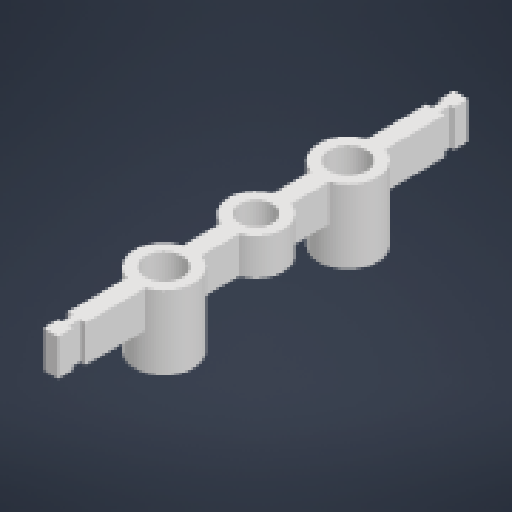
# Autodesk Inventor part: Leg_rod
Saved by Autodesk Inventor 2026 (Build 300175050, 175E)
## iProperties
Created: 2026-05-02
Part Number: Leg_rod
Material: Generic
Document SubType Name: Modeling
Designer: sniel
Density: 1 g/cm^3
Appearance: Default
Author: sniel
Autodesk Inventor part; units mm, degrees
ref_plane "YZ Plane" through (0, 0, 0) normal (1, 0, 0) x (0, 1, 0)
ref_plane "XZ Plane" through (0, 0, 0) normal (0, 1, 0) x (-1, 0, 0)
ref_plane "XY Plane" through (0, 0, 0) normal (0, 0, 1) x (1, 0, 0)
sketch "Sketch1" plane through (0, 0, 0) normal (0, 1, 0) x (-1, 0, 0)
  line L0 (16.7626, -83.8715) -> (19.7626, -83.8715) projected
  line L1 (19.7626, -83.8715) -> (19.7626, -85.3715) projected
  line L2 (19.7626, -85.3715) -> (10.7873, -88.3968) projected
  line L3 (10.7873, -88.3968) -> (7.7622, -97.3718) projected
  line L4 (7.7622, -97.3718) -> (6.2622, -97.3718) projected
  line L5 (6.2622, -97.3718) -> (6.2622, -94.3718) projected
  line L6 (6.2622, -94.3718) -> (7.2622, -94.3718) projected
  line L7 (7.2622, -94.3718) -> (7.2622, -90.3718) projected
  line L8 (7.2622, -90.3718) -> (3.2622, -90.3718) projected
  line L9 (3.2622, -90.3718) -> (3.2622, -94.3718) projected
  line L10 (3.2622, -94.3718) -> (4.2622, -94.3718) projected
  line L11 (4.2622, -94.3718) -> (4.2622, -97.3718) projected
  line L12 (4.2622, -97.3718) -> (2.7622, -97.3718) projected
  line L13 (2.7622, -97.3718) -> (-1.3715, -85.1077) projected
  arc A0 (7.4979, -76.2381) -> (-1.3715, -85.1077) centre (5.2622, -82.8718) ccw projected
  line L14 (7.4979, -76.2381) -> (19.7626, -80.3715) projected
  line L15 (19.7626, -80.3715) -> (19.7626, -81.8715) projected
  line L16 (19.7626, -81.8715) -> (16.7626, -81.8715) projected
  line L17 (16.7626, -81.8715) -> (16.7626, -80.8715) projected
  line L18 (16.7626, -80.8715) -> (12.7626, -80.8715) projected
  line L19 (12.7626, -80.8715) -> (12.7626, -84.8715) projected
  line L20 (12.7626, -84.8715) -> (16.7626, -84.8715) projected
  line L21 (16.7626, -84.8715) -> (16.7626, -83.8715) projected
  line L22 (6.3619, -198.0335) -> (6.3619, -195.0335) projected
  line L23 (6.3619, -195.0335) -> (7.8619, -195.0335) projected
  line L24 (7.8619, -195.0335) -> (10.8872, -204.0087) projected
  line L25 (10.8872, -204.0087) -> (19.8622, -207.0338) projected
  line L26 (19.8622, -207.0338) -> (19.8622, -208.5338) projected
  line L27 (19.8622, -208.5338) -> (16.8622, -208.5338) projected
  line L28 (16.8622, -208.5338) -> (16.8622, -207.5338) projected
  line L29 (16.8622, -207.5338) -> (12.8622, -207.5338) projected
  line L30 (12.8622, -207.5338) -> (12.8622, -211.5338) projected
  line L31 (12.8622, -211.5338) -> (16.8622, -211.5338) projected
  line L32 (16.8622, -211.5338) -> (16.8622, -210.5338) projected
  line L33 (16.8622, -210.5338) -> (19.8622, -210.5338) projected
  line L34 (19.8622, -210.5338) -> (19.8622, -212.0338) projected
  line L35 (19.8622, -212.0338) -> (7.5981, -216.1675) projected
  arc A1 (-1.2715, -207.2981) -> (7.5981, -216.1675) centre (5.3622, -209.5338) ccw projected
  line L36 (-1.2715, -207.2981) -> (2.8619, -195.0335) projected
  line L37 (2.8619, -195.0335) -> (4.3619, -195.0335) projected
  line L38 (4.3619, -195.0335) -> (4.3619, -198.0335) projected
  line L39 (4.3619, -198.0335) -> (3.3619, -198.0335) projected
  line L40 (3.3619, -198.0335) -> (3.3619, -202.0335) projected
  line L41 (3.3619, -202.0335) -> (7.3619, -202.0335) projected
  line L42 (7.3619, -202.0335) -> (7.3619, -198.0335) projected
  line L43 (7.3619, -198.0335) -> (6.3619, -198.0335) projected
  line L44 (2.7622, -97.3718) -> (2.8619, -195.0335)
  line L45 (7.8619, -195.0335) -> (7.7622, -97.3718)
  line L46 (2.812, -146.2026) -> (7.812, -146.2026)
  circle A2 centre (5.312, -146.2026) radius 4.5
  circle A3 centre (5.312, -146.2026) radius 7.5
  point P0 (0, 0)
  point P1 (7.8048, -139.129)
  point P2 (2.8048, -139.1341)
  point P3 (2.8193, -153.2762)
  point P4 (7.8193, -153.2711)
  dimension "d8" = 9
  dimension "d9" = 15
  constraints: 6 end point, 3 midpoint, 2 centre point, 1 coincident, 1 parallel
  measures "d8" diameter of A2
  measures "d9" diameter of A3
extrude "Extrusion1" add sketch "Sketch1" along normal blind 10 contours L45 A3 L44 L12 L11 L10 L9 L8 L7 L6 L5 L4 | A3 L45 A2 | L45 A2 L44 A3 | L44 A2 A3 | A3 L44 A2 L45 | L45 L23 L22 L43 L42 L41 L40 L39 L38 L37 L44 A3
sketch "Sketch2" plane through (0, 0, 0) normal (0, -1, 0) x (1, 0, 0)
  line L0 (-4.3619, -198.0335) -> (-3.3619, -198.0335)
  line L1 (-4.3619, -195.0335) -> (-4.3619, -198.0335)
  line L2 (-2.8619, -195.0335) -> (-4.3619, -195.0335)
  line L3 (-2.7622, -97.3718) -> (-2.8619, -195.0335)
  line L4 (-4.2622, -97.3718) -> (-2.7622, -97.3718)
  line L5 (-4.2622, -94.3718) -> (-4.2622, -97.3718)
  line L6 (-3.2622, -94.3718) -> (-4.2622, -94.3718)
  line L7 (-3.2622, -90.3718) -> (-3.2622, -94.3718)
  line L8 (-7.2622, -90.3718) -> (-3.2622, -90.3718)
  line L9 (-7.2622, -94.3718) -> (-7.2622, -90.3718)
  line L10 (-6.2622, -94.3718) -> (-7.2622, -94.3718)
  line L11 (-6.2622, -97.3718) -> (-6.2622, -94.3718)
  line L12 (-7.7622, -97.3718) -> (-6.2622, -97.3718)
  line L13 (-7.8619, -195.0335) -> (-7.7622, -97.3718)
  line L14 (-6.3619, -195.0335) -> (-7.8619, -195.0335)
  line L15 (-6.3619, -198.0335) -> (-6.3619, -195.0335)
  line L16 (-7.3619, -198.0335) -> (-6.3619, -198.0335)
  line L17 (-7.3619, -202.0335) -> (-7.3619, -198.0335)
  line L18 (-3.3619, -202.0335) -> (-7.3619, -202.0335)
  line L19 (-3.3619, -198.0335) -> (-3.3619, -202.0335)
  line L20 (-7.812, -146.2026) -> (-2.812, -146.2026)
  line L21 (-6.2622, -97.3718) -> (-4.2622, -97.3718)
  line L22 (-5.312, -146.2026) -> (-5.312, -121.2026)
  line L23 (-5.312, -146.2026) -> (-5.312, -171.2026)
  circle A0 centre (-5.312, -171.2026) radius 8
  circle A1 centre (-5.312, -121.2026) radius 8
  point P0 (0, 0)
  dimension "d2" = 25
  dimension "d3" = 25
  dimension "d4" = 16
  dimension "d5" = 16
  constraints: 48 end point, 3 midpoint, 2 centre point, 2 coincident, 2 vertical, 1 horizontal
  measures "d2" distance of L22.start L22.end
  measures "d3" distance of L22.start L23.end
  measures "d4" diameter of A0
  measures "d5" diameter of A1
extrude "Extrusion2" add sketch "Sketch2" along normal mid plane 20 contours A0 L13 L3 | L3 A0 | A0 L13 | A1 L13 L3 | L3 A1 | A1 L13
sketch "Sketch3" plane through (-5.312, -10, -121.2026) normal (0, -1, 0) x (1, 0, 0)
  circle A0 centre (0, 0) radius 8 projected
  circle A1 centre (0, -50) radius 8 projected
  circle A2 centre (0, 0) radius 5
  circle A3 centre (0, -50) radius 5
  point P0 (5.312, 121.2026)
  dimension "d10" = 10
  constraints: 2 centre point, 2 coincident
  measures "d10" diameter of A3
extrude "Extrusion3" cut sketch "Sketch3" against normal blind 20 contours A2 | A3
body "Solid1"
